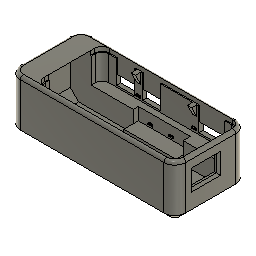
open_pill (Autodesk Fusion 360 design; units mm, degrees)
Autodesk Fusion 360 part; units mm, degrees
sketch "Sketch1" plane through (0, 0, 0) normal (0, 0, 1) x (1, 0, 0)
  line L0 (-26.5, 17.25) -> (26.5, 17.25)
  line L1 (-29.5, 17.25) -> (-39.5, 17.25)
  line L2 (-26.5, 17.25) -> (-29.5, 17.25)
  arc A0 (-39.5, 17.25) -> (-44.75, 12) centre (-39.5, 12) ccw
  line L3 (-44.75, 12) -> (-44.75, -12)
  arc A1 (-44.75, -12) -> (-39.5, -17.25) centre (-39.5, -12) ccw
  line L4 (-29.5, -17.25) -> (-39.5, -17.25)
  line L5 (-29.5, -17.25) -> (-26.35, -17.25)
  line L6 (25.75, -17.25) -> (-26.35, -17.25)
  line L7 (25.75, -17.25) -> (29.5, -17.25)
  arc A2 (29.5, -17.25) -> (34.75, -12) centre (29.5, -12) ccw
  line L8 (34.75, -12) -> (34.75, -9)
  line L9 (34.75, 9) -> (34.75, -9)
  line L10 (34.75, 9) -> (34.75, 12)
  arc A3 (34.75, 12) -> (29.5, 17.25) centre (29.5, 12) ccw
  line L11 (29.5, 17.25) -> (26.5, 17.25)
  line L12 (-26.5, 15.25) -> (26.5, 15.25)
  line L13 (-26.5, 15.25) -> (-29.5, 15.25)
  line L14 (-29.5, 15.25) -> (-39.5, 15.25)
  arc A4 (-39.5, 15.25) -> (-42.75, 12) centre (-39.5, 12) ccw
  line L15 (-42.75, 12) -> (-42.75, -12)
  arc A5 (-42.75, -12) -> (-39.5, -15.25) centre (-39.5, -12) ccw
  line L16 (-29.5, -15.25) -> (-39.5, -15.25)
  line L17 (-29.5, -15.25) -> (-26.35, -15.25)
  line L18 (25.75, -15.25) -> (-26.35, -15.25)
  line L19 (25.75, -15.25) -> (29.5, -15.25)
  arc A6 (29.5, -15.25) -> (32.75, -12) centre (29.5, -12) ccw
  line L20 (32.75, -12) -> (32.75, -9)
  line L21 (32.75, 9) -> (32.75, -9)
  line L22 (32.75, 9) -> (32.75, 12)
  arc A7 (32.75, 12) -> (29.5, 15.25) centre (29.5, 12) ccw
  line L23 (29.5, 15.25) -> (26.5, 15.25)
  dimension "d38" = 10
  constraint parallel L12 L23
  constraint perpendicular L12 L21
  constraint parallel L8 L20
  constraint parallel L9 L21
  constraint parallel L0 L12
  constraint parallel L2 L13
  constraint parallel L5 L17
  constraint parallel L6 L18
  constraint parallel L7 L19
  constraint tangent L7 A2
  constraint tangent A3 L11
  constraint tangent L10 A3
  constraint tangent A2 L8
  constraint parallel L1 L2
  constraint parallel L13 L14
  constraint parallel L4 L5
  constraint coincident A0.centre A4.centre
  constraint coincident A1.centre A5.centre
  constraint tangent L15 A5
  constraint tangent L3 A1
  measures "d38" distance of L4.start A1.end
extrude "Extrude1" add sketch "Sketch1" along normal blind 11 contours L12 L13 L14 A4 L15 A5 L16 L17 L18 L19 A6 L20 L21 L22 A7 L23 makes body 1
extrude "Extrude2" add sketch "Sketch1" along normal blind 25 bodies 1
sketch "Sketch2" plane through (0, 0, 11) normal (0, 0, 1) x (-1, 0, 0)
  line L0 (-32.75, 12) -> (-32.75, -12)
  arc A0 (-32.75, -12) -> (-29.5, -15.25) centre (-29.5, -12) ccw
  line L1 (-29.5, -15.25) -> (39.5, -15.25)
  arc A1 (39.5, -15.25) -> (42.75, -12) centre (39.5, -12) ccw
  line L2 (42.75, -12) -> (42.75, 12)
  arc A2 (42.75, 12) -> (39.5, 15.25) centre (39.5, 12) ccw
  line L3 (39.5, 15.25) -> (-29.5, 15.25)
  arc A3 (-29.5, 15.25) -> (-32.75, 12) centre (-29.5, 12) ccw
  circle A4 centre (-2, 0) radius 4.75
extrude "Extrude3" cut sketch "Sketch2" against normal up to surface (11 mm away) contours A4 bodies 1
sketch "Sketch3" plane through (0, 0, 11) normal (0, 0, 1) x (-1, 0, 0)
  circle A0 centre (-2, 0) radius 4.75
  line L0 (-32.75, 12) -> (-32.75, -12)
  arc A1 (-32.75, -12) -> (-29.5, -15.25) centre (-29.5, -12) ccw
  line L1 (-29.5, -15.25) -> (39.5, -15.25)
  arc A2 (39.5, -15.25) -> (42.75, -12) centre (39.5, -12) ccw
  line L2 (42.75, -12) -> (42.75, 12)
  arc A3 (42.75, 12) -> (39.5, 15.25) centre (39.5, 12) ccw
  line L3 (39.5, 15.25) -> (-29.5, 15.25)
  arc A4 (-29.5, 15.25) -> (-32.75, 12) centre (-29.5, 12) ccw
  line L4 (12.5, -5.5) -> (12.5, 5.5)
  line L5 (-12.5, -5.5) -> (12.5, -5.5)
  line L6 (-12.5, 5.5) -> (-12.5, -5.5)
  line L7 (12.5, 5.5) -> (-12.5, 5.5)
extrude "Extrude4" cut sketch "Sketch3" against normal blind 9 contours L4 L5 L6 L7 bodies 1
sketch "Sketch4" plane through (0, 0, 11) normal (0, 0, 1) x (-1, 0, 0)
  line L0 (-12.5, -5.5) -> (-12.5, 5.5)
  line L1 (-12.5, 5.5) -> (12.5, 5.5)
  line L2 (12.5, 5.5) -> (12.5, -5.5)
  line L3 (12.5, -5.5) -> (-12.5, -5.5)
  line L4 (-32.75, 12) -> (-32.75, -12)
  arc A0 (-32.75, -12) -> (-29.5, -15.25) centre (-29.5, -12) ccw
  line L5 (-29.5, -15.25) -> (39.5, -15.25)
  arc A1 (39.5, -15.25) -> (42.75, -12) centre (39.5, -12) ccw
  line L6 (42.75, -12) -> (42.75, 12)
  arc A2 (42.75, 12) -> (39.5, 15.25) centre (39.5, 12) ccw
  line L7 (39.5, 15.25) -> (-29.5, 15.25)
  arc A3 (-29.5, 15.25) -> (-32.75, 12) centre (-29.5, 12) ccw
  line L8 (12.5, 5.5) -> (12.5, 12.5)
  line L9 (6.5, 5.5) -> (12.5, 5.5)
  line L10 (6.5, 12.5) -> (6.5, 5.5)
  line L11 (12.5, 12.5) -> (6.5, 12.5)
extrude "Extrude5" cut sketch "Sketch4" against normal blind 7.5 contours L1 L8 L9 L10 L11 bodies 1
sketch "Sketch5" plane through (0, 0, 11) normal (0, 0, 1) x (-1, 0, 0)
  line L0 (-32.75, 12) -> (-32.75, -12)
  arc A0 (-32.75, -12) -> (-29.5, -15.25) centre (-29.5, -12) ccw
  line L1 (-29.5, -15.25) -> (39.5, -15.25)
  arc A1 (39.5, -15.25) -> (42.75, -12) centre (39.5, -12) ccw
  line L2 (42.75, -12) -> (42.75, 12)
  arc A2 (42.75, 12) -> (39.5, 15.25) centre (39.5, 12) ccw
  line L3 (39.5, 15.25) -> (-29.5, 15.25)
  arc A3 (-29.5, 15.25) -> (-32.75, 12) centre (-29.5, 12) ccw
  line L4 (6.5, 5.5) -> (6.5, 12.5)
  line L5 (6.5, 12.5) -> (12.5, 12.5)
  line L6 (12.5, 12.5) -> (12.5, -5.5)
  line L7 (12.5, -5.5) -> (-12.5, -5.5)
  line L8 (-12.5, -5.5) -> (-12.5, 5.5)
  line L9 (-12.5, 5.5) -> (6.5, 5.5)
  line L10 (12.5, -12.5) -> (12.5, -5.5)
  line L11 (-12.5, -12.5) -> (12.5, -12.5)
  line L12 (-12.5, -9) -> (-12.5, -12.5)
  line L13 (-44.75, -9) -> (-12.5, -9)
  line L14 (-32.75, -9) -> (-32.75, 9)
  line L15 (-26.5, 9) -> (-44.75, 9)
  line L16 (12.5, -5.5) -> (-12.5, -5.5)
  line L17 (-12.5, -5.5) -> (-12.5, 5.5)
  line L18 (-12.5, 5.5) -> (6.5, 5.5)
  line L19 (6.5, 5.5) -> (6.5, 12.5)
  line L20 (6.5, 12.5) -> (-12.5, 12.5)
  line L21 (-12.5, 12.5) -> (-12.5, 9.25)
  line L22 (-12.5, 9.25) -> (-26.5, 9.25)
  line L23 (-26.5, 9.25) -> (-26.5, 9)
  constraint coincident L14.start L13
  constraint coincident L14.end L15
  constraint perpendicular L14 L15
extrude "Extrude6" cut sketch "Sketch5" against normal blind 6 contours L0 L4 L7 L8 L9 L10 L11 L12 L13 L14 L15 L16 L17 L18 L19 L20 L21 L22 L23 bodies 1
sketch "Sketch6" plane through (0, 0, 11) normal (0, 0, 1) x (-1, 0, 0)
  line L0 (-12.5, -9) -> (-32.75, -9)
  line L1 (-32.75, -9) -> (-32.75, -12)
  arc A0 (-32.75, -12) -> (-29.5, -15.25) centre (-29.5, -12) ccw
  line L2 (-29.5, -15.25) -> (39.5, -15.25)
  arc A1 (39.5, -15.25) -> (42.75, -12) centre (39.5, -12) ccw
  line L3 (42.75, -12) -> (42.75, 12)
  arc A2 (42.75, 12) -> (39.5, 15.25) centre (39.5, 12) ccw
  line L4 (39.5, 15.25) -> (-29.5, 15.25)
  arc A3 (-29.5, 15.25) -> (-32.75, 12) centre (-29.5, 12) ccw
  line L5 (-32.75, 12) -> (-32.75, 9)
  line L6 (-32.75, 9) -> (-26.5, 9)
  line L7 (-26.5, 9) -> (-26.5, 9.25)
  line L8 (-26.5, 9.25) -> (-12.5, 9.25)
  line L9 (-12.5, 9.25) -> (-12.5, 12.5)
  line L10 (-12.5, 12.5) -> (12.5, 12.5)
  line L11 (12.5, 12.5) -> (12.5, -12.5)
  line L12 (12.5, -12.5) -> (-12.5, -12.5)
  line L13 (-12.5, -12.5) -> (-12.5, -9)
  line L14 (12.5, 9.25) -> (26.5, 9.25)
  line L15 (26.5, 9.25) -> (26.5, 15.25)
  line L16 (26.5, 15.25) -> (-26.5, 15.25)
  line L17 (-26.5, 15.25) -> (-26.5, 9.25)
  line L18 (-26.5, 9.25) -> (-12.5, 9.25)
  line L19 (-12.5, 9.25) -> (-12.5, 12.5)
  line L20 (-12.5, 12.5) -> (12.5, 12.5)
  line L21 (12.5, 12.5) -> (12.5, 9.25)
extrude "Extrude7" cut sketch "Sketch6" against normal blind 3 contours L4 L8 L9 L10 L11 L14 L15 L16 L17 L18 L19 L20 L21 bodies 1
sketch "Sketch7" plane through (0, 0, 11) normal (0, 0, 1) x (-1, 0, 0)
  line L0 (26.5, 15.25) -> (26.5, 9.25)
  line L1 (26.5, 9.25) -> (12.5, 9.25)
  line L2 (12.5, 9.25) -> (12.5, -12.5)
  line L3 (12.5, -12.5) -> (-12.5, -12.5)
  line L4 (-12.5, -12.5) -> (-12.5, -9)
  line L5 (-12.5, -9) -> (-32.75, -9)
  line L6 (-32.75, -9) -> (-32.75, -12)
  arc A0 (-32.75, -12) -> (-29.5, -15.25) centre (-29.5, -12) ccw
  line L7 (-29.5, -15.25) -> (39.5, -15.25)
  arc A1 (39.5, -15.25) -> (42.75, -12) centre (39.5, -12) ccw
  line L8 (42.75, -12) -> (42.75, 12)
  arc A2 (42.75, 12) -> (39.5, 15.25) centre (39.5, 12) ccw
  line L9 (39.5, 15.25) -> (26.5, 15.25)
  arc A3 (29.5, -15.25) -> (32.75, -12) centre (29.5, -12) ccw
  line L10 (32.75, -12) -> (32.75, 12)
  arc A4 (32.75, 12) -> (29.5, 15.25) centre (29.5, 12) ccw
  line L11 (32.75, 12) -> (32.75, 8) construction
  line L12 (32.75, -12) -> (32.75, -8) construction
  line L13 (32.75, -8) -> (42.75, -8)
  line L14 (32.75, 8) -> (42.75, 8)
  constraint parallel L10 L11
  constraint parallel L10 L12
  constraint coincident L8 L13.end
  constraint perpendicular L8 L13
  constraint perpendicular L10 L14
extrude "Extrude8" add sketch "Sketch7" along normal up to surface (14 mm away) contours L8 A2 L9 L10 A4 L14 | L7 A1 L8 A3 L10 L13 bodies 1
ref_plane "WorkPlane1" through (-5, 0, 11.8) normal (0, 0, 1) x (1, 0, 0)
sketch "Sketch8" plane through (-5, 0, 11.8) normal (0, 0, 1) x (1, 0, 0)
  line L0 (34.5, 15.25) -> (-24.5, 15.25) construction
  line L1 (-24.5, 15.25) -> (-20.75, 15.25) construction
  line L2 (-20.75, 15.25) -> (-12.25, 15.25)
  line L3 (-12.25, 15.25) -> (-12.25, 17.25)
  line L4 (-12.25, 17.25) -> (-20.75, 17.25)
  line L5 (-20.75, 17.25) -> (-20.75, 15.25)
  point P0 (-24.5, 15.25)
  dimension "d22" = 3.75
  dimension "d23" = 8.5
  dimension "d24" = 2
  constraint coincident P0 L0.end
  constraint parallel L0 L1
  constraint horizontal L2
  constraint vertical L3
  constraint horizontal L4
  constraint vertical L5
  measures "d22" distance of P0 L1.end
  measures "d23" distance of L1.end L2.end
  measures "d24" distance of L1.end L4.end
extrude "Extrude9" cut sketch "Sketch8" along normal blind 4.2 bodies 1
sketch "Sketch9" plane through (0, 0, 11.8) normal (0, 0, 1) x (-1, 0, 0)
  line L0 (25.75, -17.25) -> (25.75, -15.25)
  line L1 (25.75, -15.25) -> (17.25, -15.25)
  line L2 (17.25, -15.25) -> (17.25, -17.25)
  line L3 (17.25, -17.25) -> (25.75, -17.25)
  line L4 (17.25, -15.25) -> (13.15, -15.25) construction
  line L5 (13.15, -15.25) -> (4.65, -15.25)
  line L6 (4.65, -15.25) -> (4.65, -17.25)
  line L7 (4.65, -17.25) -> (13.15, -17.25)
  line L8 (13.15, -17.25) -> (13.15, -15.25)
  dimension "d73" = 3.5
  dimension "d74" = 3.5
  constraint coincident L1.end L2.start
  constraint perpendicular L2 L4
  constraint horizontal L5
  constraint vertical L6
  constraint horizontal L7
  constraint vertical L8
  measures "d27" distance of L1.end L4.end
  measures "d28" distance of L4.end L5.end
  measures "d29" distance of L4.end L7.end
extrude "Extrude10" cut sketch "Sketch9" along normal blind 4.2 contours L5 L6 L7 L8 bodies 1
sketch "Sketch10" plane through (0, 0, 11.8) normal (0, 0, 1) x (-1, 0, 0)
  line L0 (13.15, -17.25) -> (13.15, -15.25)
  line L1 (13.15, -15.25) -> (4.65, -15.25)
  line L2 (4.65, -15.25) -> (4.65, -17.25)
  line L3 (4.65, -17.25) -> (13.15, -17.25)
  line L4 (4.65, -15.25) -> (-13.85, -15.25) construction
  line L5 (-13.85, -15.25) -> (-26.35, -15.25)
  line L6 (-26.35, -15.25) -> (-26.35, -17.25)
  line L7 (-26.35, -17.25) -> (-13.85, -17.25)
  line L8 (-13.85, -17.25) -> (-13.85, -15.25)
  dimension "d32" = 18.5
  dimension "d33" = 12.5
  dimension "d34" = 2
  constraint coincident L1.end L2.start
  constraint perpendicular L2 L4
  constraint horizontal L5
  constraint vertical L6
  constraint horizontal L7
  constraint vertical L8
  measures "d32" distance of L1.end L4.end
  measures "d33" distance of L4.end L5.end
  measures "d34" distance of L4.end L7.end
extrude "Extrude11" cut sketch "Sketch10" along normal blind 4.2 contours L5 L6 L7 L8 bodies 1
chamfer "Chamfer1" distance 3 angle 45 1 edges at (32.75, 0, 5) on bodies 1
ref_plane "WorkPlane2" through (-5, 0, 11.8) normal (0, 0, 1) x (1, 0, 0)
sketch "Sketch11" plane through (-5, 0, 11.8) normal (0, 0, 1) x (1, 0, 0)
  line L0 (34.5, -15.25) -> (-24.5, -15.25) construction
  line L1 (34.5, -15.25) -> (34.5, -8.25) construction
  line L2 (37.75, -9) -> (37.75, 9) construction
  line L3 (34.5, -8.25) -> (37.75, -8.25) construction
  line L4 (37.75, -8.25) -> (39.75, -8.25)
  line L5 (39.75, -8.25) -> (39.75, 3.75)
  line L6 (39.75, 3.75) -> (37.75, 3.75)
  line L7 (37.75, 3.75) -> (37.75, -8.25)
  point P0 (34.5, -15.25)
  dimension "d42" = 7
  dimension "d43" = 2
  dimension "d44" = 12
  constraint coincident P0 L0.start
  constraint perpendicular L0 L1
  constraint horizontal L3
  constraint coincident L2 L3.end
  constraint horizontal L4
  constraint vertical L5
  constraint horizontal L6
  constraint vertical L7
  measures "d42" distance of P0 L1.end
  measures "d43" distance of L3.end L4.end
  measures "d44" distance of L3.end L6.end
extrude "Extrude12" cut sketch "Sketch11" along normal blind 2 bodies 1
extrude "Extrude13" cut 1 faces at (-36.0833, -8, 15.6667) along direction (0, -1, 0) blind 2 on bodies 1 bodies 1
extrude "Extrude14" cut 1 faces at (-36.0833, 8, 15.6667) along direction (0, 1, 0) blind 2 on bodies 1 bodies 1
sketch "Sketch12" plane through (0, 0, 11) normal (0, 0, 1) x (-1, 0, 0)
  arc A0 (29.5, -15.25) -> (32.75, -12) centre (29.5, -12) ccw
  line L0 (32.75, -12) -> (32.75, -10)
  line L1 (32.75, -10) -> (42.75, -10)
  line L2 (42.75, -10) -> (42.75, 10)
  line L3 (42.75, 10) -> (32.75, 10)
  line L4 (32.75, 10) -> (32.75, 12)
  arc A1 (32.75, 12) -> (29.5, 15.25) centre (29.5, 12) ccw
  line L5 (29.5, 15.25) -> (26.5, 15.25)
  line L6 (26.5, 15.25) -> (26.5, 9.25)
  line L7 (26.5, 9.25) -> (12.5, 9.25)
  line L8 (12.5, 9.25) -> (12.5, -12.5)
  line L9 (12.5, -12.5) -> (-12.5, -12.5)
  line L10 (-12.5, -12.5) -> (-12.5, -9)
  line L11 (-12.5, -9) -> (-32.75, -9)
  line L12 (-32.75, -9) -> (-32.75, -12)
  arc A2 (-32.75, -12) -> (-29.5, -15.25) centre (-29.5, -12) ccw
  line L13 (-29.5, -15.25) -> (29.5, -15.25)
  line L14 (32.75, -10) -> (12.5, -10)
  line L15 (12.5, 12.5) -> (12.5, 5.5)
  line L16 (32.75, 10) -> (12.5, 10)
  dimension "d51" = 180
  constraint horizontal L14
  constraint coincident L0.end L1.start
  constraint coincident L8 L14.end
  constraint coincident L3.end L4.start
  constraint coincident L15 L16.end
  measures "d51" angle of L14 L16
extrude "Extrude15" cut sketch "Sketch12" against normal up to surface (6 mm away) contours L1 L2 L3 L6 L7 L8 L14 L15 L16 bodies 1
extrude "Extrude18" add 1 faces at (-27.25, 0, 0) along direction (0, 0, -1) blind 1 on bodies 1 bodies 1
chamfer "Chamfer6" distance 3.5 distance2 3.5 8 edges at (-5, 17.25, -1) (33.2123, 15.7123, -1) (34.75, 0, -1) (33.2123, -15.7123, -1) (-5, -17.25, -1) (-43.2123, -15.7123, -1) (-44.75, 0, -1) (-43.2123, 15.7123, -1) measured on face at (-27.25, 0, -1) measured on face at (-27.25, 0, -1) measured on face at (-27.25, 0, -1) measured on face at (-27.25, 0, -1) measured on face at (-27.25, 0, -1) measured on face at (-27.25, 0, -1) measured on face at (-27.25, 0, -1) measured on face at (-27.25, 0, -1) on bodies 1
chamfer "Chamfer7" distance 1.5 distance2 1.5 1 edges at (6.4286, 1.7177, -1) measured on face at (-27.25, 0, -1) on bodies 1
sketch "Sketch15" plane through (0, 0, 25) normal (0, 0, 1) x (-1, 0, 0)
  line L0 (-34.75, 12) -> (-34.75, -12)
  arc A0 (-34.75, -12) -> (-29.5, -17.25) centre (-29.5, -12) ccw
  line L1 (-29.5, -17.25) -> (39.5, -17.25)
  arc A1 (39.5, -17.25) -> (44.75, -12) centre (39.5, -12) ccw
  line L2 (44.75, -12) -> (44.75, 12)
  arc A2 (44.75, 12) -> (39.5, 17.25) centre (39.5, 12) ccw
  line L3 (39.5, 17.25) -> (-29.5, 17.25)
  arc A3 (-29.5, 17.25) -> (-34.75, 12) centre (-29.5, 12) ccw
  line L4 (42.75, 10) -> (42.75, -10)
  line L5 (42.75, -10) -> (32.75, -10)
  line L6 (32.75, -10) -> (32.75, -12)
  arc A4 (29.5, -15.25) -> (32.75, -12) centre (29.5, -12) ccw
  line L7 (29.5, -15.25) -> (-29.5, -15.25)
  arc A5 (-32.75, -12) -> (-29.5, -15.25) centre (-29.5, -12) ccw
  line L8 (-32.75, -12) -> (-32.75, 12)
  arc A6 (-29.5, 15.25) -> (-32.75, 12) centre (-29.5, 12) ccw
  line L9 (-29.5, 15.25) -> (29.5, 15.25)
  arc A7 (32.75, 12) -> (29.5, 15.25) centre (29.5, 12) ccw
  line L10 (32.75, 12) -> (32.75, 10)
  line L11 (32.75, 10) -> (42.75, 10)
  line L12 (33.25, -10) -> (33.25, -12)
  arc A8 (29.5, -15.75) -> (33.25, -12) centre (29.5, -12) ccw
  line L13 (29.5, -15.75) -> (-29.5, -15.75)
  arc A9 (-33.25, -12) -> (-29.5, -15.75) centre (-29.5, -12) ccw
  line L14 (-33.25, -12) -> (-33.25, 12)
  arc A10 (-29.5, 15.75) -> (-33.25, 12) centre (-29.5, 12) ccw
  line L15 (-29.5, 15.75) -> (29.5, 15.75)
  arc A11 (33.25, 12) -> (29.5, 15.75) centre (29.5, 12) ccw
  line L16 (33.25, 12) -> (33.25, 10)
  dimension "d77" = -0.5
extrude "Extrude19" cut sketch "Sketch15" against normal blind 2 contours L5 L6 A4 L7 A5 L8 A6 L9 A7 L10 L11 L12 A8 L13 A9 L14 A10 L15 A11 L16 bodies 1
sketch "Sketch16" plane through (0, 0, 23) normal (0, 0, 1) x (-1, 0, 0)
  arc A0 (-29.5, 15.75) -> (-33.25, 12) centre (-29.5, 12) ccw
  line L0 (-33.25, 12) -> (-33.25, -12)
  arc A1 (-33.25, -12) -> (-29.5, -15.75) centre (-29.5, -12) ccw
  line L1 (-29.5, -15.75) -> (29.5, -15.75)
  arc A2 (29.5, -15.75) -> (33.25, -12) centre (29.5, -12) ccw
  line L2 (33.25, -12) -> (33.25, -10)
  line L3 (33.25, -10) -> (32.75, -10)
  line L4 (32.75, -10) -> (32.75, -12)
  arc A3 (29.5, -15.25) -> (32.75, -12) centre (29.5, -12) ccw
  line L5 (29.5, -15.25) -> (-29.5, -15.25)
  arc A4 (-32.75, -12) -> (-29.5, -15.25) centre (-29.5, -12) ccw
  line L6 (-32.75, -12) -> (-32.75, 12)
  arc A5 (-29.5, 15.25) -> (-32.75, 12) centre (-29.5, 12) ccw
  line L7 (-29.5, 15.25) -> (29.5, 15.25)
  arc A6 (32.75, 12) -> (29.5, 15.25) centre (29.5, 12) ccw
  line L8 (32.75, 12) -> (32.75, 10)
  line L9 (32.75, 10) -> (33.25, 10)
  line L10 (33.25, 10) -> (33.25, 12)
  arc A7 (33.25, 12) -> (29.5, 15.75) centre (29.5, 12) ccw
  line L11 (29.5, 15.75) -> (-29.5, 15.75)
  line L12 (25.75, -15.75) -> (17.25, -15.75)
  line L13 (17.25, -15.75) -> (17.25, -15.25)
  line L14 (17.25, -15.25) -> (25.75, -15.25)
  line L15 (25.75, -15.25) -> (25.75, -15.75)
  line L16 (13.15, -15.75) -> (4.65, -15.75)
  line L17 (4.65, -15.75) -> (4.65, -15.25)
  line L18 (4.65, -15.25) -> (13.15, -15.25)
  line L19 (13.15, -15.25) -> (13.15, -15.75)
  line L20 (-13.85, -15.75) -> (-26.35, -15.75)
  line L21 (-26.35, -15.75) -> (-26.35, -15.25)
  line L22 (-26.35, -15.25) -> (-13.85, -15.25)
  line L23 (-13.85, -15.25) -> (-13.85, -15.75)
  point P0 (17.25, -15.25)
  point P1 (4.65, -15.25)
  point P2 (-26.35, -15.25)
  constraint horizontal L12
  constraint vertical L13
  constraint horizontal L14
  constraint vertical L15
  constraint coincident P0 L13.end
  constraint coincident L1 L12.start
  constraint horizontal L16
  constraint vertical L17
  constraint horizontal L18
  constraint vertical L19
  constraint coincident P1 L17.end
  constraint coincident L1 L16.start
  constraint horizontal L20
  constraint vertical L21
  constraint horizontal L22
  constraint vertical L23
  constraint coincident P2 L21.end
  constraint coincident L1 L20.start
extrude "Extrude20" cut sketch "Sketch16" against normal up to surface (11.2 mm away) contours L1 L5 L20 L21 L22 L23 | L1 L5 L16 L17 L18 L19 | L1 L5 L12 L13 L14 L15 bodies 1
sketch "Sketch17" plane through (0, 10, 0) normal (0, -1, 0) x (1, 0, 0)
  line L0 (-32.75, 23) -> (-33.25, 23)
  line L1 (-33.25, 23) -> (-33.25, 25)
  line L2 (-33.25, 25) -> (-42.75, 25)
  line L3 (-42.75, 25) -> (-42.75, 5)
  line L4 (-42.75, 5) -> (-12.5, 5)
  line L5 (-12.5, 5) -> (-12.5, 11)
  line L6 (-12.5, 11) -> (-32.75, 11)
  line L7 (-32.75, 11) -> (-32.75, 23)
  line L8 (-33.25, 25) -> (-42.75, 15.5)
  line L9 (-33.25, 25) -> (-19.815, 25) construction
  dimension "d82" = 135
  constraint horizontal L9
  constraint coincident L1.end L2.start
  constraint coincident L3 L8.end
  measures "d82" angle of L8 L9
extrude "Extrude21" add sketch "Sketch17" along normal up to surface (20 mm away) contours L2 L3 L8 bodies 1
fillet "Fillet2" radius 1.5 8 edges at (-5, -17.25, 25) (33.2123, -15.7123, 25) (34.75, 0, 25) (33.2123, 15.7123, 25) (-5, 17.25, 25) (-43.2123, 15.7123, 25) (-44.75, 0, 25) (-43.2123, -15.7123, 25) on bodies 1
sketch "Sketch25" plane through (0, 0, 5) normal (0, 0, 1) x (-1, 0, 0)
  line L0 (-29.75, 9) -> (-29.75, -9)
  line L1 (-29.75, -9) -> (-12.5, -9)
  line L2 (-12.5, -9) -> (-12.5, -12.5)
  line L3 (-12.5, -12.5) -> (12.5, -12.5)
  line L4 (12.5, -12.5) -> (12.5, -10)
  line L5 (12.5, -10) -> (42.75, -10)
  line L6 (42.75, -10) -> (42.75, 10)
  line L7 (42.75, 10) -> (26.5, 10)
  line L8 (26.5, 10) -> (26.5, 9.25)
  line L9 (26.5, 9.25) -> (12.5, 9.25)
  line L10 (12.5, 9.25) -> (12.5, -5.5)
  line L11 (12.5, -5.5) -> (-12.5, -5.5)
  line L12 (-12.5, -5.5) -> (-12.5, 5.5)
  line L13 (-12.5, 5.5) -> (6.5, 5.5)
  line L14 (6.5, 5.5) -> (6.5, 12.5)
  line L15 (6.5, 12.5) -> (-12.5, 12.5)
  line L16 (-12.5, 12.5) -> (-12.5, 9.25)
  line L17 (-12.5, 9.25) -> (-26.5, 9.25)
  line L18 (-26.5, 9.25) -> (-26.5, 9)
  line L19 (-26.5, 9) -> (-29.75, 9)
  line L20 (12.5, -10) -> (12.5, -5.5)
  constraint coincident L4.end L5.start
  constraint coincident L10.end L11.start
extrude "Extrude24" cut sketch "Sketch25" against normal blind 4 contours L5 L6 L7 L8 L9 L10 L20 bodies 1
chamfer "Chamfer8" distance 4 angle 45 1 edges at (-42.75, 0, 1) on bodies 1
sketch "Sketch26" plane through (0, 0, 5) normal (0, 0, 1) x (-1, 0, 0)
  line L0 (12.5, -10) -> (12.5, -5.5)
  line L1 (12.5, -5.5) -> (-12.5, -5.5)
  line L2 (-12.5, -5.5) -> (-12.5, 5.5)
  line L3 (-12.5, 5.5) -> (6.5, 5.5)
  line L4 (6.5, 5.5) -> (6.5, 12.5)
  line L5 (6.5, 12.5) -> (-12.5, 12.5)
  line L6 (-12.5, 12.5) -> (-12.5, 9.25)
  line L7 (-12.5, 9.25) -> (-26.5, 9.25)
  line L8 (-26.5, 9.25) -> (-26.5, 9)
  line L9 (-26.5, 9) -> (-29.75, 9)
  line L10 (-29.75, 9) -> (-29.75, -9)
  line L11 (-29.75, -9) -> (-12.5, -9)
  line L12 (-12.5, -9) -> (-12.5, -12.5)
  line L13 (-12.5, -12.5) -> (12.5, -12.5)
  line L14 (12.5, -12.5) -> (12.5, -10)
  line L15 (-12.5, -9) -> (-12.5, -5.5)
  line L16 (-12.5, 5.5) -> (-12.5, 9.25)
  constraint coincident L11.end L12.start
  constraint coincident L1.end L2.start
  constraint coincident L2.end L3.start
  constraint coincident L6.end L7.start
extrude "Extrude25" cut sketch "Sketch26" against normal up to surface (4 mm away) contours L2 L7 L8 L9 L10 L11 L15 L16 bodies 1
sketch "Sketch27" plane through (0, 15.25, 0) normal (0, -1, 0) x (1, 0, 0)
  line L0 (-17.25, 23) -> (-17.25, 11.8)
  line L1 (-17.25, 11.8) -> (-25.75, 11.8)
  line L2 (-25.75, 11.8) -> (-25.75, 23)
  line L3 (-25.75, 23) -> (-29.5, 23)
  line L4 (-29.5, 23) -> (-29.5, 11)
  line L5 (-29.5, 11) -> (29.5, 11)
  line L6 (29.5, 11) -> (29.5, 23)
  line L7 (29.5, 23) -> (26.35, 23)
  line L8 (26.35, 23) -> (26.35, 11.8)
  line L9 (26.35, 11.8) -> (13.85, 11.8)
  line L10 (13.85, 11.8) -> (13.85, 23)
  line L11 (13.85, 23) -> (-4.65, 23)
  line L12 (-4.65, 23) -> (-4.65, 11.8)
  line L13 (-4.65, 11.8) -> (-13.15, 11.8)
  line L14 (-13.15, 11.8) -> (-13.15, 23)
  line L15 (-13.15, 23) -> (-17.25, 23)
  line L16 (-17.25, 23) -> (-16.2, 23) construction
  line L17 (-16.2, 23) -> (-14.2, 23)
  line L18 (-14.2, 23) -> (-14.2, 18)
  line L19 (-14.2, 18) -> (-16.2, 18)
  line L20 (-16.2, 18) -> (-16.2, 23)
  line L21 (13.85, 23) -> (12.85, 23) construction
  line L22 (12.85, 23) -> (10.85, 23)
  line L23 (10.85, 23) -> (10.85, 18)
  line L24 (10.85, 18) -> (12.85, 18)
  line L25 (12.85, 18) -> (12.85, 23)
  dimension "d123" = 1.05
  dimension "d124" = 2
  dimension "d125" = 5
  dimension "d126" = 1
  dimension "d127" = 2
  dimension "d128" = 5
  constraint coincident L0.start L15.end
  constraint perpendicular L0 L16
  constraint horizontal L17
  constraint vertical L18
  constraint horizontal L19
  constraint vertical L20
  constraint coincident L10.end L11.start
  constraint perpendicular L10 L21
  constraint horizontal L22
  constraint vertical L23
  constraint horizontal L24
  constraint vertical L25
  measures "d123" distance of L0.start L16.end
  measures "d124" distance of L16.end L17.end
  measures "d125" distance of L16.end L19.end
  measures "d126" distance of L10.end L21.end
  measures "d127" distance of L21.end L22.end
  measures "d128" distance of L21.end L24.end
extrude "Extrude26" add sketch "Sketch27" along normal blind 2.5 contours L15 L17 L18 L19 L20 | L11 L22 L23 L24 L25 bodies 1
sketch "Sketch28" plane through (-14.2, 0, 0) normal (1, 0, 0) x (0, 1, 0)
  line L0 (15.25, 18) -> (15.25, 23)
  line L1 (15.25, 23) -> (12.75, 23)
  line L2 (12.75, 23) -> (12.75, 18)
  line L3 (12.75, 18) -> (15.25, 18)
  line L4 (15.25, 18) -> (12.75, 23)
  constraint coincident L0.start L3.end
  constraint coincident L1.end L2.start
extrude "Extrude27" cut sketch "Sketch28" against normal blind 2 contours L2 L3 L4 bodies 1
sketch "Sketch29" plane through (12.85, 0, 0) normal (1, 0, 0) x (0, 1, 0)
  line L0 (15.25, 18) -> (15.25, 23)
  line L1 (15.25, 23) -> (12.75, 23)
  line L2 (12.75, 23) -> (12.75, 18)
  line L3 (12.75, 18) -> (15.25, 18)
  line L4 (15.25, 18) -> (12.75, 23)
  constraint coincident L0.start L3.end
  constraint coincident L1.end L2.start
extrude "Extrude28" cut sketch "Sketch29" against normal blind 2 contours L2 L3 L4 bodies 1
extrude "Extrude29" cut 1 faces at (33.4167, -0.25, 11.8) along direction (0, 0, -1) blind 1 on bodies 1 bodies 1
extrude "Extrude30" cut 1 faces at (33.4167, -0.25, 13.8) along direction (0, 0, 1) blind 5 on bodies 1 bodies 1
sketch "Sketch36" plane through (0, -15.25, 0) normal (0, 1, 0) x (-1, 0, 0)
  line L0 (29.5, 23) -> (-29.5, 23)
  line L1 (-29.5, 23) -> (-29.5, 11)
  line L2 (-29.5, 11) -> (-26.5, 11)
  line L3 (-26.5, 11) -> (-26.5, 8)
  line L4 (-26.5, 8) -> (26.5, 8)
  line L5 (26.5, 8) -> (26.5, 11)
  line L6 (26.5, 11) -> (29.5, 11)
  line L7 (29.5, 11) -> (29.5, 23)
  line L8 (-26.5, 11) -> (-18.5, 11) construction
  line L9 (26.5, 11) -> (18.5, 11) construction
  line L10 (-18.5, 11) -> (-18.5, 12.2) construction
  line L11 (18.5, 11) -> (18.5, 12.2) construction
  line L12 (-18.5, 12.2) -> (-16.5, 12.2)
  line L13 (-16.5, 12.2) -> (-16.5, 13.2)
  line L14 (-16.5, 13.2) -> (-18.5, 13.2)
  line L15 (-18.5, 13.2) -> (-18.5, 12.2)
  line L16 (18.5, 12.2) -> (16.5, 12.2)
  line L17 (16.5, 12.2) -> (16.5, 13.2)
  line L18 (16.5, 13.2) -> (18.5, 13.2)
  line L19 (18.5, 13.2) -> (18.5, 12.2)
  dimension "d169" = 1.2
  dimension "d170" = 1.2
  dimension "d171" = 2
  dimension "d172" = 1
  dimension "d173" = 2
  dimension "d174" = 1
  constraint horizontal L8
  constraint coincident L2.end L3.start
  constraint horizontal L9
  constraint coincident L5.end L6.start
  constraint vertical L10
  constraint vertical L11
  constraint horizontal L12
  constraint vertical L13
  constraint horizontal L14
  constraint vertical L15
  constraint horizontal L16
  constraint vertical L17
  constraint horizontal L18
  constraint vertical L19
  measures "d169" distance of L8.end L10.end
  measures "d170" distance of L9.end L11.end
  measures "d171" distance of L10.end L12.end
  measures "d172" distance of L10.end L14.end
  measures "d173" distance of L11.end L16.end
  measures "d174" distance of L11.end L18.end
extrude "Extrude31" add sketch "Sketch36" along normal blind 0.5 contours L12 L13 L14 L15 | L16 L17 L18 L19 bodies 1
chamfer "Chamfer11" distance 0.25 angle 45 4 edges at (17.5, -14.75, 13.2) (17.5, -14.75, 12.2) (-17.5, -14.75, 13.2) (-17.5, -14.75, 12.2) on bodies 1
chamfer "Chamfer12" distance 1 angle 45 4 edges at (34.75, -2.25, 18.8) (34.75, -8.25, 14.8) (34.75, -2.25, 10.8) (34.75, 3.75, 14.8) on bodies 1
sketch "Sketch37" plane through (0, 15.25, 0) normal (0, -1, 0) x (1, 0, 0)
  line L0 (10.85, 18) -> (10.85, 23)
  line L1 (10.85, 23) -> (-4.65, 23)
  line L2 (-4.65, 23) -> (-4.65, 11.8)
  line L3 (-4.65, 11.8) -> (-13.15, 11.8)
  line L4 (-13.15, 11.8) -> (-13.15, 23)
  line L5 (-13.15, 23) -> (-14.2, 23)
  line L6 (-14.2, 23) -> (-14.2, 18)
  line L7 (-14.2, 18) -> (-16.2, 18)
  line L8 (-16.2, 18) -> (-16.2, 23)
  line L9 (-16.2, 23) -> (-17.25, 23)
  line L10 (-17.25, 23) -> (-17.25, 11.8)
  line L11 (-17.25, 11.8) -> (-25.75, 11.8)
  line L12 (-25.75, 11.8) -> (-25.75, 23)
  line L13 (-25.75, 23) -> (-29.5, 23)
  line L14 (-29.5, 23) -> (-29.5, 11)
  line L15 (-29.5, 11) -> (29.5, 11)
  line L16 (29.5, 11) -> (29.5, 23)
  line L17 (29.5, 23) -> (26.35, 23)
  line L18 (26.35, 23) -> (26.35, 11.8)
  line L19 (26.35, 11.8) -> (13.85, 11.8)
  line L20 (13.85, 11.8) -> (13.85, 23)
  line L21 (13.85, 23) -> (12.85, 23)
  line L22 (12.85, 23) -> (12.85, 18)
  line L23 (12.85, 18) -> (10.85, 18)
  line L24 (-14.2, 18) -> (-14.2, 13.2) construction
  line L25 (12.85, 18) -> (12.85, 13.2) construction
  line L26 (-14.2, 13.2) -> (-16.2, 13.2)
  line L27 (-16.2, 13.2) -> (-16.2, 12.2)
  line L28 (-16.2, 12.2) -> (-14.2, 12.2)
  line L29 (-14.2, 12.2) -> (-14.2, 13.2)
  line L30 (12.85, 13.2) -> (10.85, 13.2)
  line L31 (10.85, 13.2) -> (10.85, 12.2)
  line L32 (10.85, 12.2) -> (12.85, 12.2)
  line L33 (12.85, 12.2) -> (12.85, 13.2)
  dimension "d179" = 4.8
  dimension "d180" = 4.8
  dimension "d181" = 2
  dimension "d182" = 1
  dimension "d183" = 2
  dimension "d184" = 1
  constraint coincident L6.end L7.start
  constraint perpendicular L7 L24
  constraint coincident L22.end L23.start
  constraint perpendicular L23 L25
  constraint horizontal L26
  constraint vertical L27
  constraint horizontal L28
  constraint vertical L29
  constraint horizontal L30
  constraint vertical L31
  constraint horizontal L32
  constraint vertical L33
  measures "d179" distance of L6.end L24.end
  measures "d180" distance of L22.end L25.end
  measures "d181" distance of L24.end L26.end
  measures "d182" distance of L24.end L28.end
  measures "d183" distance of L25.end L30.end
  measures "d184" distance of L25.end L32.end
extrude "Extrude32" add sketch "Sketch37" along normal blind 0.5 contours L26 L27 L28 L29 | L30 L31 L32 L33 bodies 1
chamfer "Chamfer13" distance 0.25 angle 45 4 edges at (-15.2, 14.75, 13.2) (-15.2, 14.75, 12.2) (11.85, 14.75, 13.2) (11.85, 14.75, 12.2) on bodies 1
sketch "Sketch38" plane through (0, 12.5, 0) normal (0, -1, 0) x (1, 0, 0)
  line L0 (12.5, 11) -> (-12.5, 11)
  line L1 (-12.5, 11) -> (-12.5, 5)
  line L2 (-12.5, 5) -> (12.5, 5)
  line L3 (12.5, 5) -> (12.5, 11)
  line L4 (-12.5, 5) -> (-12.5, 6) construction
  line L5 (-12.5, 6) -> (-7.5, 6) construction
  line L6 (-7.5, 6) -> (2.5, 6) construction
  line L7 (-7.5, 6) -> (-5.5, 6)
  line L8 (-5.5, 6) -> (-5.5, 7)
  line L9 (-5.5, 7) -> (-7.5, 7)
  line L10 (-7.5, 7) -> (-7.5, 6)
  line L11 (2.5, 6) -> (4.5, 6)
  line L12 (4.5, 6) -> (4.5, 7)
  line L13 (4.5, 7) -> (2.5, 7)
  line L14 (2.5, 7) -> (2.5, 6)
  dimension "d188" = 1
  dimension "d189" = 5
  dimension "d190" = 10
  dimension "d191" = 2
  dimension "d192" = 1
  dimension "d193" = 2
  dimension "d194" = 1
  constraint coincident L1.end L2.start
  constraint perpendicular L2 L4
  constraint perpendicular L4 L5
  constraint parallel L5 L6
  constraint horizontal L7
  constraint vertical L8
  constraint horizontal L9
  constraint vertical L10
  constraint horizontal L11
  constraint vertical L12
  constraint horizontal L13
  constraint vertical L14
  measures "d188" distance of L1.end L4.end
  measures "d189" distance of L4.end L5.end
  measures "d190" distance of L5.end L6.end
  measures "d191" distance of L5.end L7.end
  measures "d192" distance of L5.end L9.end
  measures "d193" distance of L6.end L11.end
  measures "d194" distance of L6.end L13.end
extrude "Extrude33" add sketch "Sketch38" along normal blind 0.5 contours L7 L8 L9 L10 | L11 L12 L13 L14 bodies 1
chamfer "Chamfer14" distance 0.25 angle 45 4 edges at (-6.5, 12, 6) (-6.5, 12, 7) (3.5, 12, 6) (3.5, 12, 7) on bodies 1
sketch "Sketch39" plane through (0, -12.5, 0) normal (0, 1, 0) x (-1, 0, 0)
  line L0 (12.5, 8) -> (-12.5, 8)
  line L1 (-12.5, 8) -> (-12.5, 5)
  line L2 (-12.5, 5) -> (6.5, 5)
  line L3 (6.5, 5) -> (6.5, 3.5)
  line L4 (6.5, 3.5) -> (12.5, 3.5)
  line L5 (12.5, 3.5) -> (12.5, 8)
  line L6 (12.5, 3.5) -> (12.5, 6) construction
  line L7 (12.5, 6) -> (7.5, 6) construction
  line L8 (7.5, 6) -> (-2.5, 6) construction
  line L9 (7.5, 6) -> (5.5, 6)
  line L10 (5.5, 6) -> (5.5, 7)
  line L11 (5.5, 7) -> (7.5, 7)
  line L12 (7.5, 7) -> (7.5, 6)
  line L13 (-2.5, 6) -> (-4.5, 6)
  line L14 (-4.5, 6) -> (-4.5, 7)
  line L15 (-4.5, 7) -> (-2.5, 7)
  line L16 (-2.5, 7) -> (-2.5, 6)
  dimension "d198" = 2.5
  dimension "d199" = 5
  dimension "d200" = 10
  dimension "d201" = 2
  dimension "d202" = 1
  dimension "d203" = 2
  dimension "d204" = 1
  constraint coincident L4.end L5.start
  constraint perpendicular L4 L6
  constraint perpendicular L6 L7
  constraint parallel L7 L8
  constraint horizontal L9
  constraint vertical L10
  constraint horizontal L11
  constraint vertical L12
  constraint horizontal L13
  constraint vertical L14
  constraint horizontal L15
  constraint vertical L16
  measures "d198" distance of L4.end L6.end
  measures "d199" distance of L6.end L7.end
  measures "d200" distance of L7.end L8.end
  measures "d201" distance of L7.end L9.end
  measures "d202" distance of L7.end L11.end
  measures "d203" distance of L8.end L13.end
  measures "d204" distance of L8.end L15.end
extrude "Extrude34" add sketch "Sketch39" along normal blind 0.5 contours L9 L10 L11 L12 | L13 L14 L15 L16 bodies 1
chamfer "Chamfer15" distance 0.25 angle 45 4 edges at (-6.5, -12, 7) (-6.5, -12, 6) (3.5, -12, 7) (3.5, -12, 6) on bodies 1
sketch "Sketch45" plane through (0, 0, -1) normal (0, 0, -1) x (1, 0, 0)
  line L0 (-39.5, -13.75) -> (29.5, -13.75)
  arc A0 (29.5, -13.75) -> (31.25, -12) centre (29.5, -12) ccw
  line L1 (31.25, -12) -> (31.25, 12)
  arc A1 (31.25, 12) -> (29.5, 13.75) centre (29.5, 12) ccw
  line L2 (29.5, 13.75) -> (-39.5, 13.75)
  arc A2 (-39.5, 13.75) -> (-41.25, 12) centre (-39.5, 12) ccw
  line L3 (-41.25, 12) -> (-41.25, -12)
  arc A3 (-41.25, -12) -> (-39.5, -13.75) centre (-39.5, -12) ccw
  circle A4 centre (2, 0) radius 6.25
  line L4 (-33.25, -10) -> (-33.25, 10) construction
  line L5 (-30.3236, 4.3851) -> (-15.3236, 4.3851) construction
  line L6 (-15.3236, 4.3851) -> (-15.3236, -3.6149) construction
  line L7 (-30.3236, 4.3851) -> (-30.3236, -3.6149) construction
  arc A5 (-30.3236, 4.3851) -> (-30.3236, -3.6149) centre (-30.3236, 0.3851) ccw
  arc A6 (-15.3236, -3.6149) -> (-15.3236, 4.3851) centre (-15.3236, 0.3851) ccw
  line L8 (-15.3236, 4.3851) -> (-30.3236, 4.3851)
  line L9 (-30.3236, -3.6149) -> (-15.3236, -3.6149)
  constraint perpendicular L4 L5
  constraint perpendicular L5 L6
  constraint perpendicular L5 L7
  constraint tangent L5 A5
  constraint tangent L5 A6
extrude "Extrude39" cut sketch "Sketch45" against normal blind 0.4 contours A5 A6 L8 L9 bodies 1
sketch "Sketch46" plane through (0, 0, -0.6) normal (0, 0, -1) x (1, 0, 0)
  line L0 (-30.3236, -3.6149) -> (-15.3236, -3.6149)
  arc A0 (-15.3236, -3.6149) -> (-15.3236, 4.3851) centre (-15.3236, 0.3851) ccw
  line L1 (-15.3236, 4.3851) -> (-30.3236, 4.3851)
  arc A1 (-30.3236, 4.3851) -> (-30.3236, -3.6149) centre (-30.3236, 0.3851) ccw
  arc A2 (-30.3236, 3.3851) -> (-30.3236, -2.6149) centre (-30.3236, 0.3851) ccw
  line L2 (-24.1943, 3.3851) -> (-24.1943, -2.6149)
  line L3 (-24.1943, 3.3851) -> (-30.3236, 3.3851)
  line L4 (-24.1943, -2.6149) -> (-30.3236, -2.6149)
  constraint concentric A1 A2
  constraint tangent A2 L3
  constraint tangent A2 L4
extrude "Extrude41" add sketch "Sketch46" along normal blind 0.4 separate body makes body 2
sketch "Sketch47" plane through (0, 0, -0.6) normal (0, 0, -1) x (1, 0, 0)
  line L0 (-30.3236, -3.6149) -> (-15.3236, -3.6149)
  arc A0 (-15.3236, -3.6149) -> (-15.3236, 4.3851) centre (-15.3236, 0.3851) ccw
  line L1 (-15.3236, 4.3851) -> (-30.3236, 4.3851)
  arc A1 (-30.3236, 4.3851) -> (-30.3236, -3.6149) centre (-30.3236, 0.3851) ccw
  arc A2 (-30.3236, 3.3851) -> (-30.3236, -2.6149) centre (-30.3236, 0.3851) ccw
  line L2 (-24.1943, 3.3851) -> (-30.3236, 3.3851)
  line L3 (-24.1943, 3.3851) -> (-24.1943, -2.6149)
  line L4 (-24.1943, -2.6149) -> (-30.3236, -2.6149)
  arc A3 (-30.3236, 3.3851) -> (-30.3236, -2.6149) centre (-30.3236, 0.3851) ccw
  point P0 (-24.1943, 3.3851)
  point P1 (-30.3236, 3.3851)
  point P2 (-24.1943, 3.3851)
  point P3 (-24.1943, -2.6149)
  constraint coincident P2 P0
  constraint coincident P1 A2.start
  constraint coincident P3 L3.end
  constraint coincident A2.end L4.end
extrude "Extrude42" add sketch "Sketch47" along normal blind 0.4 separate body contours A2 L2 L3 L4 A3 makes body 3
chamfer "Chamfer18" distance 0.2 distance2 0.4 4 edges at (-22.8236, -4.3851, -1) (-11.3236, -0.3851, -1) (-22.8236, 3.6149, -1) (-34.3236, -0.3851, -1) measured on face at (23.5833, 0, -1) measured on face at (23.5833, 0, -1) measured on face at (23.5833, 0, -1) measured on face at (23.5833, 0, -1) on bodies 1
chamfer "Chamfer19" distance 0.2 distance2 0.4 4 edges at (-22.8236, -4.3851, -1) (-34.3236, -0.3851, -1) (-22.8236, 3.6149, -1) (-11.3236, -0.3851, -1) measured on face at (-18.2805, 0.6149, -1) measured on face at (-18.2805, 0.6149, -1) measured on face at (-18.2805, 0.6149, -1) measured on face at (-18.2805, 0.6149, -1) on bodies 2
chamfer "Chamfer20" distance 0.2 distance2 0.4 4 edges at (-33.3236, -0.3851, -1) (-27.259, -3.3851, -1) (-27.259, 2.6149, -1) (-24.1943, -0.3851, -1) measured on face at (-18.2805, 0.6149, -1) measured on face at (-18.2805, 0.6149, -1) measured on face at (-18.2805, 0.6149, -1) measured on face at (-18.2805, 0.6149, -1) on bodies 2
chamfer "Chamfer21" distance 0.2 distance2 0.4 4 edges at (-27.259, -3.3851, -1) (-33.3236, -0.3851, -1) (-27.259, 2.6149, -1) (-24.1943, -0.3851, -1) measured on face at (-28.2805, 0.6149, -1) measured on face at (-28.2805, 0.6149, -1) measured on face at (-28.2805, 0.6149, -1) measured on face at (-28.2805, 0.6149, -1) on bodies 3
combine "Combine1" operation add target body 1 tool bodies 2 3
